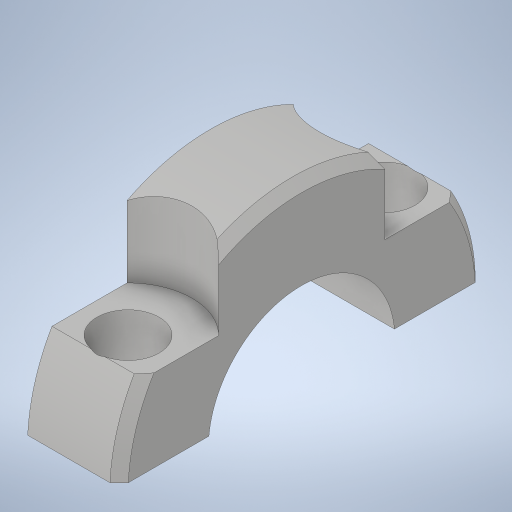
# Autodesk Inventor part: MBRDAC23-2-8_p2
Saved by Autodesk Inventor 2024 (Build 280153000, 153)
## iProperties
Created: 2024-03-05
Part Number: MBRDAC23-2-8_p2
Material: Generic
Catalog Web Link: www.cadenas.de
Description: MBRDC, MBRDAC_part2-Pulleys for Round Belts - Clamping Type - Trapezoid Groove
Vendor: MISUMI
Document SubType Name: Modeling
Designer: psAdmin
Manufacturer: MISUMI
Mass: 0.382165 g
Surface Area: 5.23666 cm^2
Volume: 0.382165 cm^3
Density: 1 g/cm^3
Appearance: PSOLRGB-175-175-175
Category: PARTsolutions
Company: MISUMI
PSOL_IDENT_0: {$CADENAS_DATA/23d-libs/misumi/metric/52_belts_pulleys/mbrdc/mbrdc_part2.prj},196 {VTYP=3D},{NB=MBRD
PSOL_IDENT_1: AC23-2-8_p2},{LINA=MBRDAC23-2-8},{NN=MBRDC, MBRDAC_part2},{DATE=06.06.2021 23:11:25},{GEOMDATE=10.06
PSOL_IDENT_2: .2016 05:41:00},{VERSION=},{LINEID=30},{WBVAR=MAT,PD,DDS},{WBNUMERIC=PD,DDS}  {NB=MBRDAC23-2-8_p2},{
PSOL_IDENT_3: LINA=MBRDAC23-2-8},{KT=DUMMY},{PN=MBRDAC23-2-8},{TYPE=MBRDAC},{MAT=2},{ST=Clear Anodizing},{AC=Hexag
PSOL_IDENT_4: on Socket Head Cap Screw (x2) Stainless Steel},{PD=23},{PD0=23,28,30,40,45,48,60,80},{U=2.0},{DDS=8.
PSOL_IDENT_5: 00},{DS0=5,6,6.35,8},{D=20},{D1=25},{D2=19},{HH=2.0},{W=4.4},{L=16},{T=10},{LL=2.5},{X=7.0},{Y=3.5},
PSOL_IDENT_6: {M=M3},{CBD=4},{MM=3.000},{MMMIN=2.459},{DD1=6.5},{DD2=3.5}
NB: MBRDAC23-2-8_p2
NN: MBRDC, MBRDAC_part2
NT: Pulleys for Round Belts - Clamping Type - Trapezoid Groove
NBSYN: $PN._p2
LINA: MBRDAC23-2-8
CATALOG: Misumi
PN: MBRDAC23-2-8
MAT: 5052 Aluminum Alloy
ST: Clear Anodizing
AC: Hexagon Socket Head Cap Screw (x2) Stainless Steel
PD: 23
U: 2
DDS: 8
D: 20
D1: 25
D2: 19
HH: 2
W: 4.4
L: 16
T: 10
LL: 2.5
X: 7
Y: 3.5
M: M3
CBD: 4
SUPPLIER: MISUMI
ARTICLENO: MBRDAC23-2-8_p2
BOMINFO: MBRDAC23-2-8
CREATOR: CADENAS GmbH
Title: MBRDAC23-2-8
Author: Cadenas PARTsolutions
Comments: Pulleys for Round Belts - Clamping Type - Trapezoid Groove
Autodesk Inventor part; units mm, degrees
sketch "Sketch_1" plane through (0, 0, 0) normal (0, 0, 1) x (1, 0, 0)
  line L0 (6, 0) -> (0, 0)
  line L1 (1, 4) -> (6, 4)
  line L2 (6, 4) -> (6, 9.5)
  line L3 (6, 9.5) -> (5.5, 10)
  line L4 (5.5, 10) -> (1, 10)
  line L5 (1, 10) -> (1, 4)
  constraints: 12 end point
revolve "Revolution1" add sketch "Sketch_1" angle 180 mid plane about axis through (6, 0, 0) along (-1, 0, 0)
sketch "Sketch_2" plane through (0, 0, 0) normal (0, 0, 1) x (1, 0, 0)
  line L0 (0, 0.5) -> (0, 0)
  line L1 (0, 0) -> (16, 0)
  line L2 (16, 0) -> (16, 0.5)
  line L3 (16, 0.5) -> (0, 0.5)
  constraints: 8 end point
extrude "Extrusion1" cut sketch "Sketch_2" along normal mid plane 40
sketch "Sketch_3" plane through (0, 0, 7) normal (0, 0, 1) x (1, 0, 0)
  line L0 (3.5, 10) -> (3.5, 0)
  line L1 (3.5, 0) -> (1.75, 0)
  line L2 (1.75, 0) -> (1.75, 3.5)
  line L3 (1.75, 3.5) -> (0.25, 3.5)
  line L4 (0.25, 3.5) -> (0.25, 10)
  line L5 (0.25, 10) -> (3.5, 10)
  line L6 (3.5, 10) -> (3.5, 0)
  constraints: 14 end point
sketch "Sketch_4" plane through (0, 0, -7) normal (0, 0, 1) x (1, 0, 0)
  line L0 (3.5, 10) -> (3.5, 0)
  line L1 (3.5, 0) -> (1.75, 0)
  line L2 (1.75, 0) -> (1.75, 3.5)
  line L3 (1.75, 3.5) -> (0.25, 3.5)
  line L4 (0.25, 3.5) -> (0.25, 10)
  line L5 (0.25, 10) -> (3.5, 10)
  line L6 (3.5, 10) -> (3.5, 0)
  constraints: 14 end point
ref_plane "part2_to_part1_XY" through (0, 0, 0) normal (1, 0, 0) x (0, 0, -1)
ref_plane "part2_to_part1_YZ" through (0, 0, 0) normal (0, 0, -1) x (0, 1, 0)
ref_plane "part2_to_part1_ZX" through (0, 0, 0) normal (0, 1, 0) x (1, 0, 0)
ref_plane "part2_to_screw1_XY" through (3.5, 3.5, 7) normal (0, 1, 0) x (1, 0, 0)
ref_plane "part2_to_screw1_YZ" through (3.5, 3.5, 7) normal (1, 0, 0) x (0, 0, -1)
ref_plane "part2_to_screw1_ZX" through (3.5, 3.5, 7) normal (0, 0, -1) x (0, 1, 0)
ref_plane "part2_to_screw2_XY" through (3.5, 3.5, -7) normal (0, 1, 0) x (1, 0, 0)
ref_plane "part2_to_screw2_YZ" through (3.5, 3.5, -7) normal (1, 0, 0) x (0, 0, -1)
ref_plane "part2_to_screw2_ZX" through (3.5, 3.5, -7) normal (0, 0, -1) x (0, 1, 0)
sketch "スケッチ7" plane through (6, 0, 0) normal (1, 0, 0) x (0, 0, -1)
  circle A0 centre (0, 0) radius 5.1
  dimension "d11" = 10.2
  constraints: 1 centre point, 1 coincident
  measures "d11" diameter of A0
extrude "押し出し4" cut sketch "スケッチ7" against normal blind 10
ref_plane "作業平面10" through (3.25, 10, 0) normal (0, 1, 0) x (-1, 0, 0)
sketch "スケッチ8" plane through (3.25, 10, 0) normal (0, 1, 0) x (-1, 0, 0)
  circle A0 centre (-0.25, 7) radius 1.75 projected
  circle A1 centre (-0.25, 7) radius 1.7
  circle A2 centre (-0.25, 7) radius 3.5
  circle A3 centre (-0.25, -7) radius 1.75 projected
  circle A4 centre (-0.25, -7) radius 1.7
  circle A5 centre (-0.25, -7) radius 3.5
  point P0 (3.25, 0)
  dimension "d14" = 3.4
  dimension "d15" = 7
  dimension "d16" = 3.4
  dimension "d17" = 7
  constraints: 4 centre point, 4 coincident
  measures "d14" diameter of A1
  measures "d15" diameter of A2
  measures "d16" diameter of A4
  measures "d17" diameter of A5
extrude "押し出し5" cut sketch "スケッチ8" against normal through all contours A1 | A4
extrude "押し出し6" cut sketch "スケッチ8" against normal blind 5 contours A0 | A1 | A2 | A3 | A4 | A5
body "Solid1"
